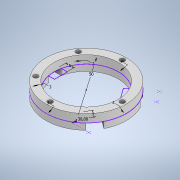
# Autodesk Inventor part: spacer
Saved by Autodesk Inventor 2021 (Build 250183000, 183)
## iProperties
Created: 2021-01-06
Part Number: spacer
Material: Generic
Document SubType Name: Modeling
Designer: awitc
Density: 1 g/cm^3
Appearance: Default
Author: awitc
Autodesk Inventor part; units mm, degrees
ref_plane "YZ Plane" through (0, 0, 0) normal (1, 0, 0) x (0, 1, 0)
ref_plane "XZ Plane" through (0, 0, 0) normal (0, 1, 0) x (-1, 0, 0)
ref_plane "XY Plane" through (0, 0, 0) normal (0, 0, 1) x (1, 0, 0)
sketch "Sketch1" plane through (0, 0, 0) normal (0, 1, 0) x (-1, 0, 0)
  circle A0 centre (0, 0) radius 25
  line L0 (22.1416, 4) -> (20.8701, 4)
  line L1 (22.1416, -4) -> (20.8701, -4)
  line L2 (24.6779, 4) -> (22.1416, 4)
  line L3 (24.6779, -4) -> (22.1416, -4)
  line L4 (-15.5618, -16.2506) -> (-14.5332, -15.5032)
  line L5 (-15.5618, 16.2506) -> (-14.5332, 15.5032)
  line L6 (-20.2641, -9.7784) -> (-19.2354, -9.0311)
  line L7 (-17.6137, -17.7414) -> (-15.5618, -16.2506)
  line L8 (-22.316, -11.2693) -> (-20.2641, -9.7784)
  line L9 (-20.2641, 9.7784) -> (-19.2354, 9.0311)
  line L10 (-17.6137, 17.7414) -> (-15.5618, 16.2506)
  line L11 (-22.316, 11.2693) -> (-20.2641, 9.7784)
  line L12 (-23.5374, 22.0452) -> (-13.679, 22.0452) construction
  arc A1 (-17.6137, -17.7414) -> (24.6779, -4) centre (0, 0) ccw
  arc A2 (24.6779, 4) -> (-17.6137, 17.7414) centre (0, 0) ccw
  arc A3 (-22.316, 11.2693) -> (-22.316, -11.2693) centre (0, 0) ccw
  line L13 (20.8701, 4) -> (15.8701, 4)
  line L14 (15.8701, 4) -> (15.8701, -4)
  line L15 (15.8701, -4) -> (20.8701, -4)
  line L16 (-14.5332, 15.5032) -> (-10.4881, 12.5643)
  line L17 (-10.4881, 12.5643) -> (-15.1903, 6.0922)
  line L18 (-15.1903, 6.0922) -> (-19.2354, 9.0311)
  line L19 (-19.2354, -9.0311) -> (-15.1903, -6.0922)
  line L20 (-15.1903, -6.0922) -> (-10.4881, -12.5643)
  line L21 (-10.4881, -12.5643) -> (-14.5332, -15.5032)
  circle A4 centre (0, 22.5) radius 1.5
  circle A5 centre (18.2029, 13.2252) radius 1.5
  circle A6 centre (18.2029, -13.2252) radius 1.5
  circle A7 centre (0, -22.5) radius 1.5
  arc A8 (-13.5023, -14.7543) -> (19.5959, -4) centre (0, 0) ccw
  arc A9 (19.5959, 4) -> (-13.5023, 14.7543) centre (0, 0) ccw
  arc A10 (-18.2046, 8.2821) -> (-18.2046, -8.2821) centre (0, 0) ccw
  circle A11 centre (-22.5, 0) radius 1.5
  circle A12 centre (0, 0) radius 20
  point P0 (-23.5374, -22.0452)
  point P1 (-28.2397, -15.5731)
  point P2 (-17.6137, 17.7414)
  point P3 (-17.6137, -17.7414)
  point P4 (24.6779, -4)
  point P5 (19.5959, -4)
  point P6 (-13.5023, 14.7543)
  dimension "d0" = 50
  dimension "d1" = 36
  dimension "d2" = 5
  dimension "d3" = 5
  dimension "d5" = 3
  dimension "d6" = 3
  dimension "d7" = 3
  dimension "d8" = 3
  dimension "d16" = 3
  constraints: 44 end point, 13 centre point, 12 point on circle, 6 point on line, 5 parallel, 4 perpendicular, 3 horizontal, 2 coincident
  measures "d0" diameter of A0
  measures "d1" angle of L10 L12
  measures "d2" distance of L15.end L15.start
  measures "d3" distance of L16.start L17.start
  measures "d5" diameter of A4
  measures "d6" diameter of A5
  measures "d7" diameter of A6
  measures "d8" diameter of A7
  measures "d16" diameter of A11
extrude "Extrusion1" add sketch "Sketch1" along normal blind 5 and the other way blind 4 contours L2 L0 L13 A9 L16 L5 L10 A0 | A0 L7 L4 L21 A8 L15 L1 L3 | L11 L9 L18 A10 L19 L6 L8 A0
extrude "Extrusion3" add sketch "Sketch1" along normal blind 5 contours A0 L3 L1 L15 A12 L13 L0 L2 | L10 L5 L16 A12 L18 L9 L11 A0 | A0 L8 L6 L19 A12 L21 L4 L7
body "Solid1"
